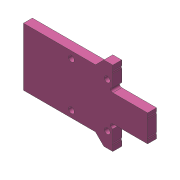
# Autodesk Inventor part: SERVO_MOUNT_TIP
Saved by Autodesk Inventor 2019.4 (Build 234330000, 330)
## iProperties
Created: 2019-11-13
Part Number: SERVO_MOUNT_TIP
Material: 一般
Document SubType Name: Modeling
Designer: y6tada
Density: 1 g/cm^3
Appearance: ピンク
Author: y6tada
Autodesk Inventor part; units mm, degrees
ref_plane "YZ Plane" through (0, 0, 0) normal (1, 0, 0) x (0, 1, 0)
ref_plane "XZ Plane" through (0, 0, 0) normal (0, 1, 0) x (-1, 0, 0)
ref_plane "XY Plane" through (0, 0, 0) normal (0, 0, 1) x (1, 0, 0)
sketch "スケッチ1" plane through (0, 0, 0) normal (0, 0, 1) x (1, 0, 0)
  line L0 (14, 10) -> (30, 10) construction
  line L1 (30, 10) -> (30, -10) construction
  line L2 (30, -10) -> (14, -10) construction
  line L3 (14, -10) -> (14, 10) construction
  line L4 (0, 0) -> (42.5052, 0) construction
  line L5 (28.5, 16.75) -> (32.5, 16.75)
  line L6 (47.1, 6) -> (47.1, 4.6)
  line L7 (32.5, -16.75) -> (28.5, -16.75)
  line L8 (32.5, 16.75) -> (32.5, 14.6)
  line L9 (32.5, 8) -> (32.5, 6) construction
  line L10 (32.5, 6) -> (47.1, 6)
  arc A0 (32.5, 8) -> (32.5, 6) centre (32.5, 7) ccw
  line L11 (32.5, -16.75) -> (32.5, -14.6)
  line L12 (32.5, -6) -> (47.1, -6)
  arc A1 (32.5, -6) -> (32.5, -8) centre (32.5, -7) ccw
  line L13 (32.5, 6) -> (32.5, -6) construction
  line L14 (32.5, -8) -> (32.5, -6) construction
  arc A2 (47.1, 4.6) -> (47.1, 3.4) centre (47.9, 4) ccw
  arc A3 (47.1, -3.4) -> (47.1, -4.6) centre (47.9, -4) ccw
  line L15 (47.1, 4.6) -> (47.1, 3.4) construction
  line L16 (47.1, 3.4) -> (47.1, -3.4)
  line L17 (47.1, -3.4) -> (47.1, -4.6) construction
  line L18 (47.1, -4.6) -> (47.1, -6)
  arc A4 (32.5, 14.6) -> (32.5, 13.4) centre (33.3, 14) ccw
  line L19 (32.5, 13.4) -> (32.5, 8)
  line L20 (32.5, 14.6) -> (32.5, 13.4) construction
  line L21 (28.5, -16.75) -> (24.75, -13)
  line L22 (24.75, -13) -> (-7.5, -13)
  line L23 (33.7, 6) -> (33.7, -6) construction
  arc A5 (32.5, -13.4) -> (32.5, -14.6) centre (33.3, -14) ccw
  line L24 (32.5, -13.4) -> (32.5, -8)
  line L25 (32.5, -14.6) -> (32.5, -13.4) construction
  line L26 (28.5, 16.75) -> (24.75, 13)
  line L27 (24.75, 13) -> (-7.5, 13)
  line L28 (-7.5, 13) -> (-7.5, -13)
  line L29 (28.5, 16.75) -> (28.5, -16.75) construction
  line L30 (35.7, 6) -> (35.7, -6) construction
  dimension "d0" = 20
  dimension "d1" = 16
  dimension "d3" = 1
  dimension "d4" = 12
  dimension "d5" = 2.5
  dimension "d7" = 1
  dimension "d8" = 0.8
  dimension "d9" = 8
  dimension "d10" = 0.8
  dimension "d11" = 28
  dimension "d12" = 33.5
  dimension "d14" = 4
  dimension "d16" = 45
  dimension "d29" = 1.2
  dimension "d31" = 3
  dimension "d32" = 40
  dimension "d34" = 32.5
  dimension "d35" = 45
  dimension "d36" = 2
  dimension "d37" = 11.4
  constraints: 62 end point, 14 perpendicular, 12 point on circle, 11 symmetric about line, 6 centre point, 5 parallel, 4 coincident, 4 horizontal, 3 point on line, 3 vertical, 1 collinear, 1 equal radius, 1 tangent, 6 other
  measures "d0" distance of L0.end L1.end
  measures "d1" distance of L0.start L0.end
  measures "d3" radius of A0
  measures "d4" diameter of L10 L4
  measures "d5" distance between parallel lines of L8 L1
  measures "d7" radius of A2
  measures "d8" distance from line of L6 A2.centre
  measures "d9" diameter of A2.centre L4
  measures "d10" distance from line of L8 A4.centre
  measures "d11" diameter of A4.centre L4
  measures "d12" distance between parallel lines of L7 L5
  measures "d14" distance of L7.start L7.end
  measures "d16" angle of L7 L21
  measures "d29" distance between parallel lines of L13 L23
  measures "d31" distance between parallel lines of L2 L22
  measures "d32" distance between parallel lines of L19 L28
  measures "d34" distance from line of L4.start L19
  measures "d35" angle of L26 L5
  measures "d36" distance between parallel lines of L23 L30
  measures "d37" distance between parallel lines of L16 L30
extrude "押し出し1" add sketch "スケッチ1" along normal blind 4
hole "穴1" at (14, 10, 0) at (30, 10, 0) at (30, -10, 0) at (14, -10, 0) direction (0, 0, 1) diameter 2.6 end through all clearance for "Countersunk Raised Head Screw ISO 2010/7047" size "M2.5" standard "ISO"
